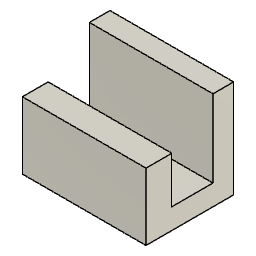
sorted_smarties_cover_connector_clip (Autodesk Fusion 360 design; units mm, degrees)
Autodesk Fusion 360 part; units mm, degrees
sketch "Sorted Smarties Cover Connector Clip" plane through (0, 0, 0) normal (0, 0, 1) x (1, 0, 0)
  line L0 (0, 0) -> (24, 0)
  line L1 (24, 0) -> (24, 17)
  line L2 (24, 17) -> (0, 17)
  line L3 (0, 17) -> (0, 0)
  dimension "d6" = 24
  dimension "d7" = 17
  constraint horizontal L0
  constraint vertical L1
  constraint horizontal L2
  constraint vertical L3
  constraint coincident L0.start L3.end
  measures "d6" distance of L0.start L0.end
  measures "d7" distance of L0.end L1.end
extrude "Extrude1" add sketch "Sorted Smarties Cover Connector Clip" along normal blind 4
sketch "Connecting Section" plane through (0, 0, 4) normal (0, 0, 1) x (-1, 0, 0)
  line L0 (0, -17) -> (0, 0)
  line L1 (0, 0) -> (-24, 0)
  line L2 (-24, 0) -> (-24, -17)
  line L3 (-24, -17) -> (0, -17)
  line L4 (0, -17) -> (-24, -17)
  line L5 (-24, -17) -> (-24, -12)
  line L6 (-24, -12) -> (0, -12)
  line L7 (0, -12) -> (0, -17)
  dimension "d5" = 5
  constraint horizontal L4
  constraint vertical L5
  constraint horizontal L6
  constraint vertical L7
  constraint coincident L2 L5.end
  constraint coincident L0.start L3.end
  measures "d5" distance of L2.end L5.end
extrude "Extrude2" add sketch "Connecting Section" along normal blind 9 contours L0 L2 L3 L4 L5 L6 L7
sketch "Sorted Smarties Cover Section" plane through (0, 0, 4) normal (0, 0, 1) x (-1, 0, 0)
  line L0 (-24, -12) -> (0, -12)
  line L1 (0, -12) -> (0, 0)
  line L2 (0, 0) -> (-24, 0)
  line L3 (-24, 0) -> (-24, -12)
  line L4 (0, 0) -> (-24, 0)
  line L5 (-24, 0) -> (-24, -4)
  line L6 (-24, -4) -> (0, -4)
  line L7 (0, -4) -> (0, 0)
  dimension "d8" = 4
  constraint horizontal L4
  constraint vertical L5
  constraint horizontal L6
  constraint vertical L7
  constraint coincident L3 L5.end
  constraint coincident L1.end L2.start
  measures "d8" distance of L4 L6
extrude "Extrude3" add sketch "Sorted Smarties Cover Section" along normal blind 15 contours L1 L2 L3 L4 L5 L6 L7
move_body "Move1" bodies 1 to x (-1, 0, 0) y (0, -1, 0) z (0, 0, 1) at (24, 17, 0)
named bodies: "Sorted Smarties Cover Connector Clip"
